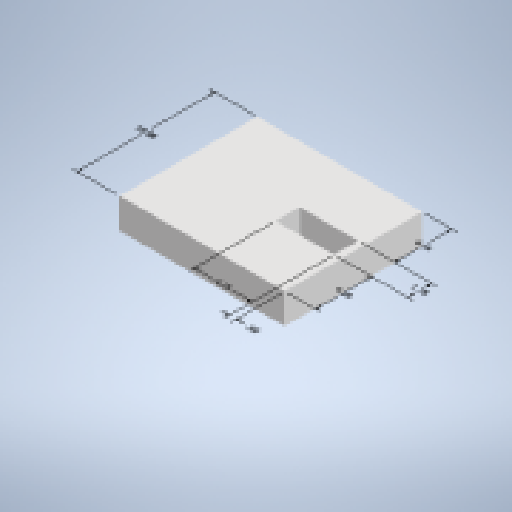
# Autodesk Inventor part: floor
Saved by Autodesk Inventor 2024 (Build 280153000, 153)
## iProperties
Created: 2023-12-28
Part Number: floor
Material: Generic
Document SubType Name: Sheet Metal
Designer: ctam0
Density: 1 g/cm^3
Appearance: Default
Sheet Metal Rule: Default
Author: ctam0
Autodesk Inventor part; units mm, degrees
ref_plane "YZ Plane" through (0, 0, 0) normal (1, 0, 0) x (0, 1, 0)
ref_plane "XZ Plane" through (0, 0, 0) normal (0, 1, 0) x (-1, 0, 0)
ref_plane "XY Plane" through (0, 0, 0) normal (0, 0, 1) x (1, 0, 0)
sketch "Sketch1" plane through (0, 0, 0) normal (0, 1, 0) x (-1, 0, 0)
  line L0 (-152.4, 127) -> (152.4, 127)
  line L1 (152.4, 127) -> (152.4, -127)
  line L2 (152.4, -127) -> (-152.4, -127)
  line L3 (-152.4, -127) -> (-152.4, 127)
  line L4 (-152.4, 127) -> (152.4, -127) construction
  line L5 (152.4, 127) -> (-152.4, -127) construction
  line L6 (-139.7, -21.3407) -> (-31.75, -21.3407)
  line L7 (-31.75, -21.3407) -> (-31.75, 23.1093)
  line L8 (-31.75, 23.1093) -> (-139.7, 23.1093)
  line L9 (-139.7, 23.1093) -> (-139.7, -21.3407)
  line L10 (-139.7, -21.3407) -> (-31.75, 23.1093) construction
  line L11 (-31.75, -21.3407) -> (-139.7, 23.1093) construction
  point P0 (0, 0)
  point P1 (-85.725, 0.8843)
  dimension "d0" = 304.8
  dimension "d1" = 254
  dimension "d2" = 107.95
  dimension "d3" = 44.45
  dimension "d4" = 12.7
  constraints: 24 end point, 4 midpoint, 4 parallel, 2 horizontal, 2 perpendicular
  measures "d0" distance of L1.end L2.end
  measures "d1" distance of L0.end L1.end
  measures "d2" distance of L8.end L7.end
  measures "d3" distance of L7.end L6.end
  measures "d4" distance between parallel lines of L3 L9
extrude "Extrusion1" add sketch "Sketch1" along normal blind 55.88
sketch "Sketch8" plane through (0, 0, 0) normal (0, -1, 0) x (1, 0, 0)
  line L0 (139.7, 23.1093) -> (31.75, 23.1093) projected
  line L1 (69.85, 23.1093) -> (101.6, 23.1093)
  line L2 (101.6, 23.1093) -> (101.6, 28.1893)
  line L3 (101.6, 28.1893) -> (69.85, 28.1893)
  line L4 (69.85, 28.1893) -> (69.85, 23.1093)
  line L5 (31.75, -21.3407) -> (139.7, -21.3407) projected
  line L6 (69.85, -21.3407) -> (101.6, -21.3407)
  line L7 (101.6, -21.3407) -> (101.6, -26.4207)
  line L8 (101.6, -26.4207) -> (69.85, -26.4207)
  line L9 (69.85, -26.4207) -> (69.85, -21.3407)
  line L10 (31.75, 23.1093) -> (31.75, -21.3407) projected
  point P0 (0, 0)
  point P1 (69.85, -23.8807)
  dimension "d47" = 31.75
  dimension "d48" = 5.08
  dimension "d49" = 38.1
  dimension "d50" = 31.75
  dimension "d51" = 5.08
  dimension "d52" = 38.1
  constraints: 16 end point, 4 parallel, 2 horizontal, 2 perpendicular, 2 point on line, 1 midpoint
  measures "d47" distance of L3.end L2.end
  measures "d48" distance of L2.end L1.end
  measures "d49" distance from line of L0.end L4
  measures "d50" distance of L7.end L8.end
  measures "d51" distance of L6.end L7.end
  measures "d52" distance from line of L10 point (69.85, -23.881)
extrude "Extrusion8" add sketch "Sketch8" along normal blind 38.1
sketch "Sketch9" plane through (139.7, 55.88, 23.1093) normal (0, 0, -1) x (-1, 0, 0)
  circle A0 centre (53.91, -74.6062) radius 6 projected
  circle A1 centre (53.91, -74.6062) radius 6
  point P0 (139.7, -55.88)
  constraints: 1 centre point, 1 coincident, 1 concentric
extrude "Extrusion9" cut sketch "Sketch9" against normal blind 38.1
sketch "Sketch10" plane through (101.6, 0, -26.4207) normal (0, 0, -1) x (-1, 0, 0)
  circle A0 centre (15.81, -18.7262) radius 6 projected
  circle A1 centre (15.81, -18.7262) radius 6
  point P0 (101.6, 0)
  constraints: 1 centre point, 1 coincident, 1 concentric
extrude "Extrusion10" cut sketch "Sketch10" against normal blind 38.1
sketch "Sketch11" plane through (0, 55.88, 0) normal (0, 1, 0) x (1, 0, 0)
  point P0 (0, 0)
equation "\"BendRadius\" = Thickness"
equation "\"BendReliefWidth\" = Thickness"
equation "\"BendReliefDepth\" = 0.5 * Thickness"
equation "\"CornerReliefSize\" = 4 * Thickness"
equation "\"MinimumRemnant\" = 2 * Thickness"
equation "\"TransitionRadius\" = BendRadius"
equation "\"JacobiRadiusSize\" = BendRadius"
equation "\"GapSize\" = Thickness"
equation "\"Thickness\" = 12.7"
body "Solid1"
